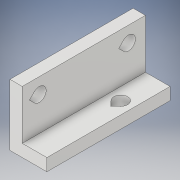
# Autodesk Inventor part: Y-axis Belt Idler 2
Saved by Autodesk Inventor 2018 (Build 220112000, 112)
## iProperties
Created: 2013-10-27
Part Number: Y-axis Belt Idler 2
Material: ASA Plastic
Document SubType Name: Modeling
Designer: Gabriel Smolnycki
Mass: 4.57544 g
Surface Area: 28.6329 cm^2
Volume: 4.27611 cm^3
Density: 1.07 g/cm^3
Appearance: Smooth - White ASA
Sending System: SolidWorks 2017
Last Author: Gabriel Smolnycki
Last Saved: 2017-09-14
Author: Gabriel Smolnycki
Autodesk Inventor part; units mm, degrees
ref_plane "YZ Plane" through (0, 0, 0) normal (1, 0, 0) x (0, 1, 0)
ref_plane "XZ Plane" through (0, 0, 0) normal (0, 1, 0) x (-1, 0, 0)
ref_plane "XY Plane" through (0, 0, 0) normal (0, 0, 1) x (1, 0, 0)
sketch "Sketch1" plane through (0, 0, 0) normal (0, 0, 1) x (1, 0, 0)
  line L0 (15, 4) -> (7, 4)
  line L1 (15, 0) -> (15, 4)
  line L2 (3, 0) -> (15, 0)
  line L3 (3, 20) -> (3, 0)
  line L4 (7, 20) -> (3, 20)
  line L5 (7, 4) -> (7, 20)
  constraints: 12 end point, 3 horizontal, 3 vertical, 1 perpendicular
extrude "Extrusion4" add sketch "Sketch1" along normal blind 40
sketch "Sketch2" plane through (7, 4, 0) normal (0, 1, 0) x (1, 0, 0)
  arc A0 (5.591, -13.591) -> (2.409, -13.591) centre (4, -12) ccw
  line L0 (4, -15.182) -> (5.591, -13.591)
  line L1 (2.409, -13.591) -> (4, -15.182)
  constraints: 4 end point, 2 perpendicular, 2 point on circle, 1 centre point
extrude "Extrusion3" cut sketch "Sketch2" against normal blind 4
sketch "Sketch3" plane through (7, 4, 0) normal (1, 0, 0) x (0, 0, -1)
  arc A0 (-7.091, 9.409) -> (-7.091, 12.591) centre (-5.5, 11) ccw
  line L0 (-8.682, 11) -> (-7.091, 9.409)
  line L1 (-7.091, 12.591) -> (-8.682, 11)
  constraints: 4 end point, 2 perpendicular, 2 point on circle, 1 centre point
extrude "Extrusion2" cut sketch "Sketch3" against normal blind 4 draft 0
sketch "Sketch4" plane through (7, 4, 0) normal (1, 0, 0) x (0, 0, -1)
  line L0 (-36.091, 12.591) -> (-37.682, 11)
  arc A0 (-36.091, 9.409) -> (-36.091, 12.591) centre (-34.5, 11) ccw
  line L1 (-37.682, 11) -> (-36.091, 9.409)
  constraints: 4 end point, 2 perpendicular, 2 point on circle, 1 centre point
extrude "Extrusion1" cut sketch "Sketch4" against normal blind 4
body "Solid3"
